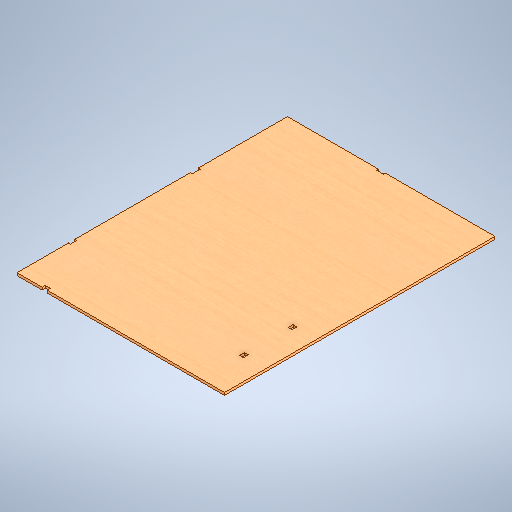
# Autodesk Inventor part: MainFloorPanel
Saved by Autodesk Inventor 2026.2 (Build 302298010, 298A)
## iProperties
Created: 2026-03-17
Part Number: MainFloorPanel
Material: Drewno (wiśnia)
Document SubType Name: Modeling
Designer: Patryk
Density: 0.63 g/cm^3
Appearance: Wiśnia — naturalna — niski połysk
Mass: 301.518 g
Surface Area: 2452.04 cm^2
Volume: 478.6 cm^3
Author: Patryk
Autodesk Inventor part; units mm, degrees
ref_plane "YZ Plane" through (0, 0, 0) normal (1, 0, 0) x (0, 1, 0)
ref_plane "XZ Plane" through (0, 0, 0) normal (0, 1, 0) x (-1, 0, 0)
ref_plane "XY Plane" through (0, 0, 0) normal (0, 0, 1) x (1, 0, 0)
sketch "Szkic1" plane through (0, 0, 0) normal (0, 1, 0) x (-1, 0, 0)
  line L0 (-165, -215) -> (165, -215)
  line L1 (165, -215) -> (165, 215)
  line L2 (165, 215) -> (-165, 215)
  line L3 (-165, 215) -> (-165, -215)
  line L4 (-165, -215) -> (165, 215) construction
  line L5 (165, -215) -> (-165, 215) construction
  point P0 (0, 0)
  dimension "d0" = 330
  dimension "d1" = 430
  constraints: 12 end point, 2 midpoint, 2 parallel, 1 horizontal, 1 perpendicular
  measures "d0" distance of L2.end L1.end
  measures "d1" distance of L1.end L0.end
extrude "Wyciągnięcie proste1" add sketch "Szkic1" along normal mid plane 4
sketch "Szkic2" plane through (0, 2, 0) normal (0, 1, 0) x (1, 0, 0)
  line L0 (165, -215) -> (165, 215) projected
  line L1 (-165, -215) -> (165, -215) projected
  line L2 (165, 215) -> (-165, 215) projected
  line L3 (-165, 215) -> (-165, -215) projected
  line L4 (-165, -133) -> (-162, -133)
  line L5 (-162, -133) -> (-162, -123)
  line L6 (-162, -123) -> (-165, -123)
  line L7 (-165, -123) -> (-165, -133)
  line L8 (-165, 61) -> (-162, 61)
  line L9 (-162, 61) -> (-162, 73)
  line L10 (-162, 73) -> (-165, 73)
  line L11 (-165, 73) -> (-165, 61)
  line L12 (-125, -215) -> (-117, -215)
  line L13 (-117, -215) -> (-117, -210)
  line L14 (-117, -210) -> (-125, -210)
  line L15 (-125, -210) -> (-125, -215)
  line L16 (132, -144) -> (126, -144)
  line L17 (126, -144) -> (126, -152)
  line L18 (126, -152) -> (132, -152)
  line L19 (132, -152) -> (132, -144)
  line L20 (132, -67) -> (126, -67)
  line L21 (126, -67) -> (126, -75)
  line L22 (126, -75) -> (132, -75)
  line L23 (132, -75) -> (132, -67)
  line L24 (-10, 215) -> (-20, 215)
  line L25 (-20, 215) -> (-20, 212)
  line L26 (-20, 212) -> (-10, 212)
  line L27 (-10, 212) -> (-10, 215)
  point P0 (0, 0)
  point P1 (-125, -212.5)
  point P2 (-165, 73)
  point P3 (-165, -123)
  point P4 (-20, 213.5)
  dimension "d23" = 82
  dimension "d24" = 10
  dimension "d25" = 3
  dimension "d26" = 12
  dimension "d27" = 3
  dimension "d29" = 8
  dimension "d30" = 40
  dimension "d31" = 5
  dimension "d38" = 276
  dimension "d39" = 63
  dimension "d40" = 6
  dimension "d41" = 33
  dimension "d42" = 8
  dimension "d43" = 140
  dimension "d44" = 8
  dimension "d45" = 33
  dimension "d46" = 6
  dimension "d49" = 145
  dimension "d50" = 10
  dimension "d51" = 3
  constraints: 48 end point, 12 parallel, 6 horizontal, 6 perpendicular, 4 point on line, 2 midpoint
  measures "d23" distance between parallel lines of L1 L4
  measures "d24" distance of L4.end L5.end
  measures "d25" distance of L4.start L4.end
  measures "d26" distance of L8.end L9.end
  measures "d27" distance of L8.start L8.end
  measures "d29" distance of L14.end L13.end
  measures "d30" distance from line of point (-125, -212.5) L3
  measures "d31" distance of L12.end L13.end
  measures "d38" distance between parallel lines of L8 L1
  measures "d39" distance between parallel lines of L1 L18
  measures "d40" distance of L16.start L16.end
  measures "d41" distance between parallel lines of L0 L19
  measures "d42" distance of L16.end L17.end
  measures "d43" distance between parallel lines of L1 L22
  measures "d44" distance of L20.end L21.end
  measures "d45" distance between parallel lines of L23 L0
  measures "d46" distance of L20.start L20.end
  measures "d49" distance from line of L3 point (-20, 213.5)
  measures "d50" distance of L25.end L26.end
  measures "d51" distance of L26.end L24.start
extrude "Wyciągnięcie proste4" cut sketch "Szkic2" against normal through all contours L1 L15 L14 L13 | L3 L6 L5 L4 | L10 L9 L8 L3
extrude "Wyciągnięcie proste5" cut sketch "Szkic2" against normal through all contours L19 L18 L17 L16 | L23 L22 L21 L20
extrude "Wyciągnięcie proste6" cut sketch "Szkic2" against normal through all contours L27 L26 L25 L2
